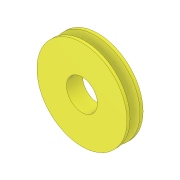
# Autodesk Inventor part: CLB_072_ScissorPulley
Saved by Autodesk Inventor 2018 (Build 220112000, 112)
## iProperties
Created: 2020-02-17
Part Number: CLB_072_ScissorPulley
Material: PC/ABS Plastic
Document SubType Name: Modeling
Designer: 22perngrac
Density: 0.357273 g/cm^3
Appearance: Smooth - Yellow
Mass: 2.40032 g
Surface Area: 63.9212 cm^2
Volume: 6.71845 cm^3
Author: 22perngrac
Autodesk Inventor part; units mm, degrees
ref_plane "YZ Plane" through (0, 0, 0) normal (1, 0, 0) x (0, 1, 0)
ref_plane "XZ Plane" through (0, 0, 0) normal (0, 1, 0) x (-1, 0, 0)
sketch "Sketch1" plane through (0, 0, 0) normal (0, 0, 1) x (1, 0, 0)
  circle A0 centre (0, 0) radius 23.0505
  dimension "d0" = 46.101
  constraints: 1 centre point, 1 coincident
  measures "d0" diameter of A0
extrude "Extrusion1" add sketch "Sketch1" along normal blind 1.5875
sketch "Sketch4" plane through (0, 0, 0) normal (0, 0, -1) x (-1, 0, 0)
  circle A0 centre (0, 0) radius 13.8303
  circle A1 centre (0, 0) radius 23.0505 projected
  dimension "d14" = 27.6606
  constraints: 1 centre point, 1 coincident
  measures "d14" diameter of A0
extrude "Extrusion2" add sketch "Sketch4" along normal blind 2.54 contours A0
ref_plane "Work Plane2" through (0, 0, -2.54) normal (0, 0, -1) x (-1, 0, 0)
mirror "Mirror1" about plane through (0, 0, -2.54) normal (0, 0, -1) of "Extrusion1", "Extrusion2"
sketch "Sketch5" plane through (0, 0, 1.5875) normal (0, 0, 1) x (1, 0, 0)
  point P0 (0, 0)
  point P1 (0, 0)
  constraints: 1 coincident
hole "Hole1" at (0, 0, 1.5875) direction (0, 0, -1) diameter 15.875 end through all
body "Solid1"
